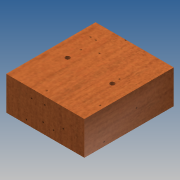
# Autodesk Inventor part: hubjig_blocks
Saved by Autodesk Inventor 2014 SP1 (Build 180222100, 222)
## iProperties
Created: 2014-08-29
Part Number: hubjig_blocks
Material: Wood (Cherry)
Document SubType Name: Modeling
Designer: Dave
Mass: 216.801 g
Surface Area: 325.806 cm^2
Volume: 344.128 cm^3
Density: 0.63 g/cm^3
Appearance: Cherry - Natural Low Gloss
Author: Dave
Autodesk Inventor part; units mm, degrees
ref_plane "YZ Plane" through (0, 0, 0) normal (1, 0, 0) x (0, 1, 0)
ref_plane "XZ Plane" through (0, 0, 0) normal (0, 1, 0) x (-1, 0, 0)
ref_plane "XY Plane" through (0, 0, 0) normal (0, 0, 1) x (1, 0, 0)
sketch "Sketch1" plane through (0, 0, 0) normal (0, 0, 1) x (1, 0, 0)
  line L0 (0, 0) -> (88.9, 0)
  line L1 (88.9, 0) -> (88.9, 38.1)
  line L2 (88.9, 38.1) -> (0, 38.1)
  line L3 (0, 38.1) -> (0, 0)
  dimension "d0" = 88.9
  dimension "d1" = 38.1
  constraints: 8 end point, 2 parallel, 1 horizontal, 1 perpendicular
  measures "d0" distance of L0.start L0.end
  measures "d1" distance of L2.end L0.start
extrude "Extrusion1" add sketch "Sketch1" along normal blind 101.6
sketch "Sketch3" plane through (0, 38.1, 0) normal (0, 1, 0) x (1, 0, 0)
  line L0 (88.9, 0) -> (0, 0) projected
  line L1 (88.9, -101.6) -> (0, -101.6) projected
  line L2 (88.9, 0) -> (88.9, -101.6) projected
  circle A0 centre (69.85, -50.8) radius 4.3006
  line L3 (44.45, 0) -> (44.45, -101.6) construction
  circle A1 centre (19.05, -50.8) radius 4.3006
  dimension "d4" = 19.05
  constraints: 2 centre point, 2 end point, 2 midpoint, 1 symmetric about line, 1 other
  measures "d4" distance from line of L2 A0.centre
hole "Hole1" at (19.05, 38.1, 50.8) at (69.85, 38.1, 50.8) direction (0, -1, 0) diameter 5.1054 end through all clearance for "Flat Head Machine Screw (82)" size "#10" standard "Ansi Unified Screw Threads"
sketch "Sketch4" plane through (0, 0, 0) normal (0, -1, 0) x (1, 0, 0)
  circle A0 centre (19.05, 50.8) radius 2.5527 projected
  circle A1 centre (69.85, 50.8) radius 2.5527 projected
  line L0 (0, 0) -> (88.9, 0) projected
  line L1 (0, 101.6) -> (88.9, 101.6) projected
  line L2 (44.45, 101.6) -> (44.45, 0) construction
  circle A2 centre (31.75, 69.85) radius 5.9334
  line L3 (19.05, 50.8) -> (69.85, 50.8) construction
  circle A3 centre (57.15, 69.85) radius 5.9334
  circle A4 centre (31.75, 31.75) radius 5.9334
  circle A5 centre (57.15, 31.75) radius 5.9334
  dimension "d12" = 19.05
  dimension "d13" = 12.7
  constraints: 4 centre point, 4 end point, 3 symmetric about line, 2 midpoint, 1 perpendicular, 3 other
  measures "d12" vertical distance of L3.start A2.centre
  measures "d13" distance from line of A2.centre L2
hole "Hole2" at (31.75, 0, 69.85) at (57.15, 0, 69.85) at (57.15, 0, 31.75) at (31.75, 0, 31.75) direction (0, 1, 0) diameter 5.1054 depth 25.4 tip angle 118 clearance for "Flat Head Machine Screw (82)" size "#10" standard "Ansi Unified Screw Threads"
body "Solid1"
